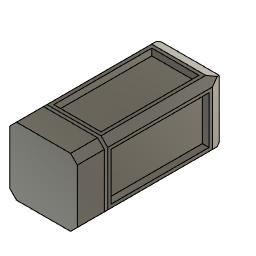
Guard2 (Autodesk Fusion 360 design; units mm, degrees)
Autodesk Fusion 360 part; units mm, degrees
sketch "Sketch1" plane through (0, 0, 0) normal (0, 0, 1) x (1, 0, 0)
  line L0 (12.7, 12.7) -> (-12.7, 12.7)
  line L1 (-12.7, 12.7) -> (-12.7, -12.7)
  line L2 (-12.7, -12.7) -> (12.7, -12.7)
  line L3 (12.7, -12.7) -> (12.7, 12.7)
  line L4 (12.7, 12.7) -> (-12.7, -12.7) construction
  line L5 (-12.7, 12.7) -> (12.7, -12.7) construction
  constraint horizontal L0
  constraint perpendicular L0 L1
  constraint parallel L0 L2
  constraint parallel L1 L3
  constraint coincident L4 origin
  constraint coincident L5 origin
extrude "Extrude1" add sketch "Sketch1" along normal blind 19.05
sketch "Sketch2" plane through (12.7, 0, 0) normal (1, 0, 0) x (0, 1, 0)
  line L0 (-12.7, 0) -> (12.7, 0)
  line L1 (12.7, 0) -> (12.7, 19.05)
  line L2 (12.7, 19.05) -> (-12.7, 19.05)
  line L3 (-12.7, 19.05) -> (-12.7, 0)
  line L4 (-12.7, 17.78) -> (-11.43, 17.78)
  line L5 (-11.43, 17.78) -> (-11.43, 16.51)
  line L6 (-11.43, 16.51) -> (-12.7, 16.51)
  line L7 (-12.7, 16.51) -> (-12.7, 17.78)
  line L8 (12.7, 17.78) -> (11.43, 17.78)
  line L9 (11.43, 17.78) -> (11.43, 16.51)
  line L10 (11.43, 16.51) -> (12.7, 16.51)
  line L11 (12.7, 16.51) -> (12.7, 17.78)
  constraint horizontal L4
  constraint vertical L5
  constraint horizontal L6
  constraint vertical L7
  constraint coincident L3 L4.start
  constraint horizontal L8
  constraint vertical L9
  constraint horizontal L10
  constraint vertical L11
  constraint coincident L1 L8.start
extrude "Extrude2" cut sketch "Sketch2" against normal blind 25.4 contours L3 L4 L5 L6 L7 | L1 L8 L9 L10 L11
sketch "Sketch3" plane through (0, -12.7, 0) normal (0, -1, 0) x (1, 0, 0)
  line L0 (12.7, 16.51) -> (-12.7, 16.51)
  line L1 (-12.7, 16.51) -> (-12.7, 0)
  line L2 (-12.7, 0) -> (12.7, 0)
  line L3 (12.7, 0) -> (12.7, 16.51)
  line L4 (-12.7, 17.78) -> (-11.43, 17.78)
  line L5 (-11.43, 17.78) -> (-11.43, 16.51)
  line L6 (-11.43, 16.51) -> (-12.7, 16.51)
  line L7 (-12.7, 16.51) -> (-12.7, 17.78)
  line L8 (12.7, 16.51) -> (11.43, 16.51)
  line L9 (11.43, 16.51) -> (11.43, 17.78)
  line L10 (11.43, 17.78) -> (12.7, 17.78)
  line L11 (12.7, 17.78) -> (12.7, 16.51)
  constraint horizontal L4
  constraint vertical L5
  constraint horizontal L6
  constraint vertical L7
  constraint horizontal L8
  constraint vertical L9
  constraint horizontal L10
  constraint vertical L11
  constraint coincident L0.start L3.end
extrude "Extrude3" cut sketch "Sketch3" against normal blind 25.4 contours L0 L8 L9 L10 L11 | L0 L4 L5 L6 L7
extrude "Extrude4" cut 1 faces at (-4.2333, 4.2333, 0) along direction (0, 0, 1) blind 6.35
extrude "Extrude5" add 1 faces at (-4.2333, 4.2333, 19.05) along direction (0, 0, 1) blind 50.8
chamfer "Chamfer1" distance 10.16 angle 45 1 edges at (-12.7, 0, 69.85)
chamfer "Chamfer2" distance 2.5375 angle 45 3 edges at (-12.7, 12.7, 38.735) (-12.7, -12.7, 38.735) (-12.7, 0, 59.69)
chamfer "Chamfer3" distance 2.5375 angle 45 4 edges at (-12.7, -12.7, 11.43) (-12.7, 12.7, 11.43) (12.7, -12.7, 11.43) (12.7, 12.7, 11.43)
chamfer "Chamfer4" distance 2.54 angle 45 4 edges at (-11.43, 11.43, 17.145) (11.43, 11.43, 17.145) (-11.43, -11.43, 17.145) (11.43, -11.43, 17.145)
chamfer "Chamfer5" distance 10.16 angle 45 1 edges at (5.08, 12.7, 69.85)
chamfer "Chamfer6" distance 10.16 angle 45 1 edges at (12.7, -5.08, 69.85)
chamfer "Chamfer7" distance 10.16 angle 45 1 edges at (0, -12.7, 69.85)
chamfer "Chamfer8" distance 2.5375 angle 45 5 edges at (1.2687, 12.7, 59.69) (12.7, 12.7, 38.735) (12.7, 0, 59.69) (12.7, -12.7, 38.735) (1.2687, -12.7, 59.69)
sketch "Sketch6" plane through (12.7, 0, 0) normal (1, 0, 0) x (0, 1, 0)
  line L0 (10.1625, 57.1525) -> (-10.1625, 57.1525)
  line L1 (-10.1625, 57.1525) -> (-10.1625, 17.78)
  line L2 (-10.1625, 17.78) -> (10.1625, 17.78)
  line L3 (10.1625, 17.78) -> (10.1625, 57.1525)
  line L4 (8.89, 55.88) -> (-8.9636, 55.88)
  line L5 (-8.9636, 55.88) -> (-8.9636, 19.0525)
  line L6 (-8.9636, 19.0525) -> (8.89, 19.0525)
  line L7 (8.89, 19.0525) -> (8.89, 55.88)
  line L8 (8.89, 55.88) -> (-8.9636, 19.0525) construction
  line L9 (-8.9636, 55.88) -> (8.89, 19.0525) construction
  point P0 (-0.0368, 37.4663)
  constraint horizontal L4
  constraint perpendicular L4 L5
  constraint parallel L4 L6
  constraint parallel L5 L7
  constraint coincident L8 P0
  constraint coincident L9 P0
extrude "Extrude6" cut sketch "Sketch6" against normal blind 2.54 contours L4 L5 L6 L7
sketch "Sketch7" plane through (0, 12.7, 0) normal (0, 1, 0) x (-1, 0, 0)
  line L0 (10.1625, 57.1525) -> (-10.1625, 57.1525)
  line L1 (-10.1625, 57.1525) -> (-10.1625, 17.78)
  line L2 (-10.1625, 17.78) -> (10.1625, 17.78)
  line L3 (10.1625, 17.78) -> (10.1625, 57.1525)
  line L4 (8.89, 55.88) -> (-8.8377, 55.88)
  line L5 (-8.8377, 55.88) -> (-8.8377, 19.0525)
  line L6 (-8.8377, 19.0525) -> (8.89, 19.0525)
  line L7 (8.89, 19.0525) -> (8.89, 55.88)
  line L8 (8.89, 55.88) -> (-8.8377, 19.0525) construction
  line L9 (-8.8377, 55.88) -> (8.89, 19.0525) construction
  point P0 (0.0262, 37.4663)
  constraint horizontal L4
  constraint perpendicular L4 L5
  constraint parallel L4 L6
  constraint parallel L5 L7
  constraint coincident L8 P0
  constraint coincident L9 P0
extrude "Extrude7" cut sketch "Sketch7" against normal blind 2.54 contours L4 L5 L6 L7
sketch "Sketch8" plane through (-12.7, 0, 0) normal (-1, 0, 0) x (0, -1, 0)
  line L0 (-10.1625, 57.1525) -> (-10.1625, 17.78)
  line L1 (-10.1625, 17.78) -> (10.1625, 17.78)
  line L2 (10.1625, 17.78) -> (10.1625, 57.1525)
  line L3 (10.1625, 57.1525) -> (-10.1625, 57.1525)
  line L4 (8.89, 55.88) -> (-8.8653, 55.88)
  line L5 (-8.8653, 55.88) -> (-8.8653, 19.0525)
  line L6 (-8.8653, 19.0525) -> (8.89, 19.0525)
  line L7 (8.89, 19.0525) -> (8.89, 55.88)
  line L8 (8.89, 55.88) -> (-8.8653, 19.0525) construction
  line L9 (-8.8653, 55.88) -> (8.89, 19.0525) construction
  point P0 (0.0123, 37.4663)
  constraint horizontal L4
  constraint perpendicular L4 L5
  constraint parallel L4 L6
  constraint parallel L5 L7
  constraint coincident L8 P0
  constraint coincident L9 P0
extrude "Extrude8" cut sketch "Sketch8" against normal blind 2.54 contours L4 L5 L6 L7
sketch "Sketch9" plane through (0, -12.7, 0) normal (0, -1, 0) x (1, 0, 0)
  line L0 (10.1625, 57.1525) -> (-10.1625, 57.1525)
  line L1 (-10.1625, 57.1525) -> (-10.1625, 17.78)
  line L2 (-10.1625, 17.78) -> (10.1625, 17.78)
  line L3 (10.1625, 17.78) -> (10.1625, 57.1525)
  line L4 (8.89, 55.88) -> (-8.8405, 55.88)
  line L5 (-8.8405, 55.88) -> (-8.8405, 19.0525)
  line L6 (-8.8405, 19.0525) -> (8.89, 19.0525)
  line L7 (8.89, 19.0525) -> (8.89, 55.88)
  line L8 (8.89, 55.88) -> (-8.8405, 19.0525) construction
  line L9 (-8.8405, 55.88) -> (8.89, 19.0525) construction
  point P0 (0.0248, 37.4663)
  constraint horizontal L4
  constraint perpendicular L4 L5
  constraint parallel L4 L6
  constraint parallel L5 L7
  constraint coincident L8 P0
  constraint coincident L9 P0
extrude "Extrude9" cut sketch "Sketch9" against normal blind 2.54 contours L4 L5 L6 L7
chamfer "Chamfer9" distance 2.5397 angle 45 4 edges at (-2.54, 0, 69.85) (0, 2.54, 69.85) (2.54, 0, 69.85) (0, -2.54, 69.85)
move_body "Move1" bodies 1 to x (1, 0, 0) y (0, 1, 0) z (0, 0, 1) at (-1.0854, 0, -6.3383)
move_body "Move2" bodies 1 to x (1, 0, 0) y (0, 0, -1) z (0, 1, 0) at (0, -31.1403, 31.1156)
move_body "Move3" bodies 1 to x (1, 0, 0) y (0, 1, 0) z (0, 0, 1) at (0, 0, -17.78)
move_body "Move4" bodies 1 to x (1, 0, 0) y (0, 1, 0) z (0, 0, 1) at (1.0922, 0, 0)
move_body "Move5" bodies 1 to x (1, 0, 0) y (0, 1, 0) z (0, 0, 1) at (0, 0, -12.7)
move_body "Move6" bodies 1 to x (1, 0, 0) y (0, 1, 0) z (0, 0, 1) at (0, 0, -0.6096)
move_body "Move7" bodies 1 to x (1, 0, 0) y (0, 1, 0) z (0, 0, 1) at (0, 31.115, 0)
